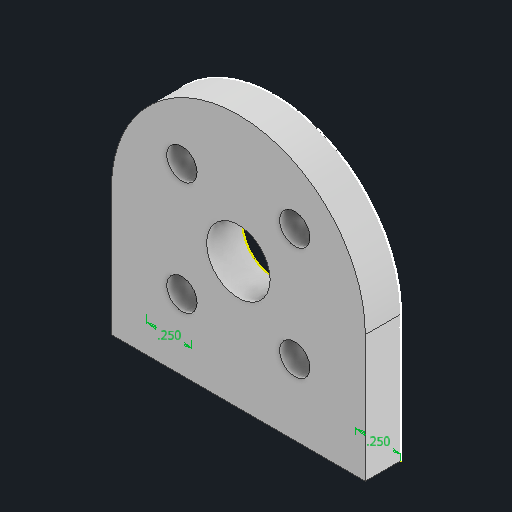
# Autodesk Inventor part: Custom GoBilda Yellow Jacket Motor Mount
Saved by Autodesk Inventor 2022 (Build 260153000, 153)
## iProperties
Created: 2021-10-09
Part Number: Custom GoBilda Yellow Jacket Motor Mount
Material: Generic
Document SubType Name: Modeling
Designer: divid
Density: 1 g/cm^3
Appearance: Default
Author: divid
Autodesk Inventor part; units mm, degrees
ref_plane "YZ Plane" through (0, 0, 0) normal (1, 0, 0) x (0, 1, 0)
ref_plane "XZ Plane" through (0, 0, 0) normal (0, 1, 0) x (-1, 0, 0)
ref_plane "XY Plane" through (0, 0, 0) normal (0, 0, 1) x (1, 0, 0)
sketch "Sketch2" plane through (0, 0, 0) normal (0, 0, 1) x (1, 0, 0)
  line L0 (0, 0) -> (0, 8) construction
  line L1 (0, 8) -> (-8, 8) construction
  line L2 (-8, 8) -> (8, 8) construction
  line L3 (8, 8) -> (8, -8) construction
  line L4 (8, -8) -> (-8, -8) construction
  line L5 (-8, -8) -> (-8, 8) construction
  circle A0 centre (-8, 8) radius 2.15
  circle A1 centre (8, 8) radius 2.15
  circle A2 centre (8, -8) radius 2.15
  circle A3 centre (-8, -8) radius 2.15
  circle A4 centre (0, 0) radius 4.5
  line L6 (18, 0) -> (18, -12.7)
  line L7 (-18, -7.4) -> (-18, 0)
  line L8 (-18, -7.4) -> (-18, -18)
  line L9 (-18, -18) -> (18, -18)
  line L10 (18, -18) -> (18, -12.7)
  arc A5 (18, 0) -> (-18, 0) centre (0, 0) ccw
  arc A6 (-18, 0) -> (18, 0) centre (0, 0) ccw construction
  point P0 (-14.1994, 16.0997)
  dimension "d0" = 8
  dimension "d1" = 8
  dimension "d2" = 16
  dimension "d3" = 16
  dimension "d4" = 4.3
  dimension "d5" = 4.3
  dimension "d6" = 4.3
  dimension "d7" = 4.3
  dimension "d8" = 9
  dimension "d13" = 18
  dimension "d15" = 18
  dimension "d16" = 18
  constraints: 22 end point, 7 centre point, 5 coincident, 4 point on circle, 3 parallel, 3 perpendicular, 2 horizontal, 2 tangent, 2 vertical
  measures "d0" distance of L0.start L0.end
  measures "d1" distance of L0.end L1.end
  measures "d2" distance of L3.end L4.end
  measures "d3" distance of L2.end L3.end
  measures "d4" diameter of A0
  measures "d5" diameter of A1
  measures "d6" diameter of A2
  measures "d7" diameter of A3
  measures "d8" diameter of A4
  measures "d13" distance from line of L6 L0.start
  measures "d15" radius of A6
  measures "d16" distance from line of L9 A6.centre
extrude "Extrusion1" add sketch "Sketch2" along normal blind 5
sketch "Sketch3" plane through (-18, -18, 0) normal (0, -1, 0) x (1, 0, 0)
  point P0 (18, 0)
sketch "Sketch4" plane through (0, 0, 0) normal (0, 0, -1) x (-1, 0, 0)
  circle A0 centre (0, 0) radius 4.5 projected
  circle A1 centre (0, 0) radius 18
  line L0 (-18, -18) -> (-18, 0) projected
  line L1 (-18, 0) -> (-18, -18)
  line L2 (18, -18) -> (-18, -18) projected
  line L3 (-18, -18) -> (18, -18)
  line L4 (18, 0) -> (18, -18) projected
  line L5 (18, 0) -> (18, -18)
  line L6 (-18, -18) -> (-11.65, -18) construction
  line L7 (-11.65, -18) -> (-11.65, -13.7214)
  line L8 (18, -18) -> (11.65, -18) construction
  line L9 (11.65, -18) -> (11.65, -13.7214)
  dimension "d17" = 6.35
  dimension "d18" = 6.35
  constraints: 14 end point, 3 point on circle, 2 collinear, 2 perpendicular, 2 point on line, 2 tangent, 1 centre point, 1 coincident, 1 vertical
  measures "d17" distance of L0.start L6.end
  measures "d18" distance of L2.start L8.end
sketch "Sketch5" plane through (-18, -18, 0) normal (0, -1, 0) x (1, 0, 0)
  point P0 (18, 0)
body "Solid1"
